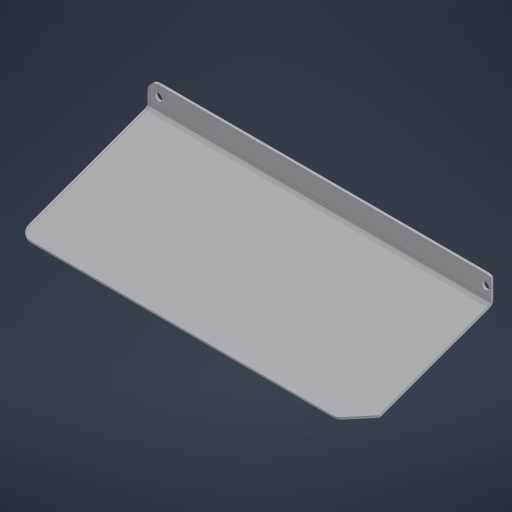
# Autodesk Inventor part: wing_wedge
Saved by Autodesk Inventor 2024 (Build 280153000, 153)
## iProperties
Created: 2024-01-16
Part Number: wing_wedge
Material: Glass, Frosted
Document SubType Name: Modeling
Designer: avere
Density: 2.18 g/cm^3
Appearance: Frosted - White
Author: avere
Autodesk Inventor part; units mm, degrees
ref_plane "YZ Plane" through (0, 0, 0) normal (1, 0, 0) x (0, 1, 0)
ref_plane "XZ Plane" through (0, 0, 0) normal (0, 1, 0) x (-1, 0, 0)
ref_plane "XY Plane" through (0, 0, 0) normal (0, 0, 1) x (1, 0, 0)
sketch "Sketch1" plane through (0, 0, 0) normal (0, 0, 1) x (1, 0, 0)
  circle A0 centre (0, 0) radius 2.1844
  arc A1 (0, 6.35) -> (-6.35, 0) centre (0, 0) ccw
  line L0 (-6.35, 0) -> (-6.35, -82.55)
  line L1 (0, -88.9) -> (176.7104, -88.9)
  line L2 (-6.351, -6.35) -> (193.5393, -6.3491)
  circle A2 centre (190.499, 0.0009) radius 2.1844
  arc A3 (193.5393, 5.5757) -> (190.4991, 6.3509) centre (190.499, 0.0009) ccw
  line L3 (192.7883, -79.044) -> (180.3526, -87.7516)
  line L4 (196.85, -76.2) -> (212.0312, -76.2) construction
  arc A4 (176.7104, -88.9) -> (180.3526, -87.7516) centre (176.7104, -82.55) ccw
  arc A5 (192.7883, -79.044) -> (193.5393, -78.4274) centre (189.1461, -73.8424) ccw
  arc A6 (-6.35, -82.55) -> (0, -88.9) centre (0, -82.55) ccw
  line L5 (165.0634, -0.0075) -> (177.7634, -0.0075) construction
  line L6 (190.4991, 6.3509) -> (182.7829, 6.3509)
  line L7 (182.7829, 6.3509) -> (0, 6.35)
  line L8 (193.5393, 5.5757) -> (193.5393, -78.4274)
  point P0 (-6.35, -88.9)
  point P1 (196.85, -88.9)
  point P2 (195.4961, -77.148)
  point P3 (196.3859, -76.2)
  point P4 (157.4407, 6.3507)
  dimension "d0" = 4.3688
  dimension "d2" = 12.7
  dimension "d4" = 88.9
  dimension "d9" = 4.3688
  dimension "d10" = 145
  dimension "d12" = 6.35
  dimension "d13" = 6.35
  dimension "d14" = 6.35
  constraints: 18 end point, 10 point on circle, 9 tangent, 7 centre point, 7 point on line, 3 coincident, 2 horizontal, 1 equal length, 1 perpendicular, 1 vertical
  measures "d0" diameter of A0
  measures "d2" diameter of A1
  measures "d4" distance of L0.start point (-6.35, -88.9)
  measures "d9" diameter of A2
  measures "d10" angle of L3 L4
  measures "d12" radius of A4
  measures "d13" radius of A5
  measures "d14" radius of A6
extrude "Extrusion1" add sketch "Sketch1" along normal blind 1.5875
bend part "Bend Part1" radius 3.175 angle 70 line through (-6.351, -6.35, 0) along (1, 0.0000048, 0) centre toward (0, 0, 1) moving side (0.0000048, -1, 0) both sides no
body "Solid1"
